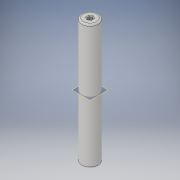
# Autodesk Inventor part: tube
Saved by Autodesk Inventor 2019 (Build 230136000, 136)
## iProperties
Created: 2018-09-29
Part Number: tube
Material: Generic
Document SubType Name: Modeling
Designer: mrhftc
Density: 1 g/cm^3
Appearance: Default
Author: mrhftc
Autodesk Inventor part; units mm, degrees
ref_plane "YZ Plane" through (0, 0, 0) normal (1, 0, 0) x (0, 1, 0)
ref_plane "XZ Plane" through (0, 0, 0) normal (0, 1, 0) x (-1, 0, 0)
ref_plane "XY Plane" through (0, 0, 0) normal (0, 0, 1) x (1, 0, 0)
sketch "Sketch3" plane through (0, 0, 0) normal (0, 1, 0) x (-1, 0, 0)
  circle A0 centre (0, 0) radius 10
  line L0 (0, 7.3639) -> (0, 0)
  line L1 (0, 0) -> (0, -8.8137)
  line L2 (6.485, 0) -> (0, 0)
  line L3 (-6.963, 0) -> (0, 0)
  line L4 (0, 3.0022) -> (2.6, 1.5011)
  line L5 (0, 3.0022) -> (3.0022, 3.0022) construction
  circle A1 centre (0, 0) radius 10
  line L6 (0, 3.0022) -> (-2.6, 1.5011)
  line L7 (0, -3.0022) -> (2.6, -1.5011)
  line L8 (0, -3.0022) -> (-2.6, -1.5011)
  line L9 (2.6, 1.5011) -> (2.6, -1.5011)
  line L10 (-2.6, 1.5011) -> (-2.6, -1.5011)
  dimension "d6" = 30
  dimension "d7" = 5.2
  dimension "d8" = 3.0022
  dimension "d9" = 3.0022
  dimension "d10" = 20
  constraints: 22 end point, 4 symmetric about line, 3 point on line, 2 centre point, 2 horizontal, 2 vertical, 1 coincident, 1 collinear, 1 equal length, 1 parallel, 1 other
  measures "d6" angle of L4 L5
  measures "d7" distance between parallel lines of L6 L7
  measures "d8" distance of L4.start L4.end
  measures "d9" distance of L4.end L7.end
  measures "d10" diameter of A0
extrude "Extrusion2" add sketch "Sketch3" along normal blind 152.4
fillet "Fillet3" radius 2 1 edges at (10, 0, 0)
fillet "Fillet4" radius 1 6 edges at (1.3, 0, -2.2517) (-1.3, 0, -2.2517) (-2.6, 0, 0) (-1.3, 0, 2.2517) (1.3, 0, 2.2517) (2.6, 0, 0)
ref_plane "Work Plane1" through (0, 76.2, 0) normal (0, -1, 0) x (1, 0, 0)
mirror "Mirror1" about plane through (0, 76.2, 0) normal (0, -1, 0) of "Fillet4", "Fillet3"
equation "\"d8\" = d9"
body "Solid2"
